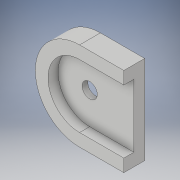
# Autodesk Inventor part: Chain Guard rear arm
Saved by Autodesk Inventor 2017 (Build 210142000, 142)
## iProperties
Created: 2019-10-23
Part Number: Chain Guard rear arm
Material: Generic
Document SubType Name: Modeling
Designer: Delta
Density: 1 g/cm^3
Appearance: Default
Author: Delta
Autodesk Inventor part; units mm, degrees
ref_plane "YZ Plane" through (0, 0, 0) normal (1, 0, 0) x (0, 1, 0)
ref_plane "XZ Plane" through (0, 0, 0) normal (0, 1, 0) x (-1, 0, 0)
ref_plane "XY Plane" through (0, 0, 0) normal (0, 0, 1) x (1, 0, 0)
sketch "Sketch1" plane through (0, 0, 0) normal (0, 0, 1) x (1, 0, 0)
  circle A0 centre (0, 0) radius 44.45
  line L0 (0, 44.45) -> (44.45, 44.45)
  line L1 (44.45, 44.45) -> (44.45, -44.45)
  line L2 (44.45, -44.45) -> (0, -44.45)
  line L3 (0, -44.45) -> (0, 44.45)
  dimension "d0" = 88.9
  dimension "d1" = 44.45
  dimension "d2" = 88.9
  constraints: 8 end point, 2 parallel, 1 coincident, 1 horizontal, 1 perpendicular, 1 vertical alignment, 2 other
  measures "d1" distance between parallel lines of L1 L3
  measures "d2" distance of L0.end L1.end
extrude "Extrusion1" add sketch "Sketch1" along normal blind 20.955
sketch "Sketch2" plane through (0, 0, 20.955) normal (0, 0, 1) x (1, 0, 0)
  arc A0 (0, 44.45) -> (0, -44.45) centre (0, 0) ccw projected
  circle A1 centre (0, 0) radius 31.75
  line L0 (44.45, 44.45) -> (44.45, -44.45) projected
  line L1 (0, 31.75) -> (44.45, 31.75)
  line L2 (44.45, 31.75) -> (44.45, -31.75)
  line L3 (44.45, -31.75) -> (0, -31.75)
  line L4 (0, -31.75) -> (0, 31.75)
  dimension "d5" = 63.5
  dimension "d6" = 63.5
  dimension "d7" = 44.45
  constraints: 8 end point, 2 parallel, 1 coincident, 1 horizontal, 1 perpendicular, 1 point on line, 1 vertical alignment, 2 other
  measures "d6" distance between parallel lines of L3 L1
  measures "d7" distance between parallel lines of L0 L4
extrude "Extrusion2" cut sketch "Sketch2" against normal blind 10.16
sketch "Sketch3" plane through (0, 0, 10.795) normal (0, 0, 1) x (1, 0, 0)
  circle A0 centre (0, 0) radius 7.62
  dimension "d10" = 15.24
  constraints: 1 centre point, 1 coincident
  measures "d10" diameter of A0
extrude "Extrusion3" cut sketch "Sketch3" against normal through all
sketch "Sketch4" plane through (0, 0, 0) normal (0, 0, -1) x (-1, 0, 0)
  circle A0 centre (0, 0) radius 15.24
  dimension "d13" = 30.48
  constraints: 1 centre point, 1 coincident
  measures "d13" diameter of A0
extrude "Extrusion4" cut sketch "Sketch4" against normal blind 5.08
equation "\"d1\" = 0.5 * d0"
equation "\"d2\" = d0"
equation "\"d6\" = d5"
body "Solid1"
